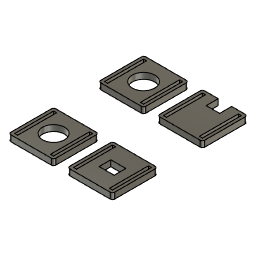
Bracelets v2 (Autodesk Fusion 360 design; units mm, degrees)
Autodesk Fusion 360 part; units mm, degrees
ref_plane "WorkPlane1" through (0, 0, 0) normal (0, 0, 1) x (1, 0, 0)
sketch "Sketch1" plane through (0, 0, 0) normal (0, 0, 1) x (1, 0, 0)
  line L0 (1.5, 0) -> (28.5, 0)
  line L1 (30, 1.5) -> (30, 28.5)
  line L2 (28.5, 30) -> (1.5, 30)
  line L3 (0, 28.5) -> (0, 1.5)
  arc A0 (30, 28.5) -> (28.5, 30) centre (28.5, 28.5) ccw
  arc A1 (1.5, 30) -> (0, 28.5) centre (1.5, 28.5) ccw
  arc A2 (0, 1.5) -> (1.5, 0) centre (1.5, 1.5) ccw
  arc A3 (28.5, 0) -> (30, 1.5) centre (28.5, 1.5) ccw
  line L4 (15, 0) -> (15, 30) construction
  line L5 (34.631, -0.4878) -> (34.631, 26.5001) construction
  line L6 (30, 15) -> (0, 15) construction
  arc A4 (40.762, 30) -> (39.262, 28.5) centre (40.762, 28.5) ccw
  line L7 (40.762, 30) -> (67.762, 30)
  arc A5 (69.262, 28.5) -> (67.762, 30) centre (67.762, 28.5) ccw
  line L8 (69.262, 28.5) -> (69.262, 1.5)
  arc A6 (67.762, 0) -> (69.262, 1.5) centre (67.762, 1.5) ccw
  line L9 (67.762, 0) -> (40.762, 0)
  arc A7 (39.262, 1.5) -> (40.762, 0) centre (40.762, 1.5) ccw
  line L10 (39.262, 1.5) -> (39.262, 28.5)
  line L11 (39.262, 15) -> (69.262, 15) construction
  line L12 (54.262, 0) -> (54.262, 30) construction
  line L13 (4, 2) -> (2, 2)
  line L14 (2, 2) -> (2, 28)
  line L15 (2, 28) -> (4, 28)
  line L16 (4, 28) -> (4, 2)
  line L17 (28, 28) -> (26, 28)
  line L18 (26, 28) -> (26, 2)
  line L19 (28, 2) -> (28, 28)
  line L20 (26, 2) -> (28, 2)
  line L21 (67.262, 28) -> (65.262, 28)
  line L22 (65.262, 28) -> (65.262, 2)
  line L23 (67.262, 2) -> (67.262, 28)
  line L24 (65.262, 2) -> (67.262, 2)
  line L25 (43.262, 28) -> (43.262, 2)
  line L26 (41.262, 2) -> (41.262, 28)
  line L27 (43.262, 2) -> (41.262, 2)
  line L28 (41.262, 28) -> (43.262, 28)
  line L29 (0, 45) -> (70, 45) construction
  line L30 (67.262, 62) -> (65.262, 62)
  line L31 (43.262, 62) -> (43.262, 88)
  line L32 (28, 88) -> (28, 62)
  arc A8 (28.5, 60) -> (30, 61.5) centre (28.5, 61.5) ccw
  line L33 (34.631, 90.4878) -> (34.631, 63.4999) construction
  line L34 (4, 88) -> (2, 88)
  line L35 (15, 90) -> (15, 60) construction
  line L36 (39.262, 75) -> (69.262, 75) construction
  arc A9 (40.762, 90) -> (39.262, 88.5) centre (40.762, 88.5) ccw
  arc A10 (30, 88.5) -> (28.5, 90) centre (28.5, 88.5) ccw
  arc A11 (67.762, 60) -> (69.262, 61.5) centre (67.762, 61.5) ccw
  line L37 (0, 61.5) -> (0, 88.5)
  line L38 (30, 88.5) -> (30, 61.5)
  line L39 (1.5, 90) -> (28.5, 90)
  arc A12 (1.5, 90) -> (0, 88.5) centre (1.5, 88.5) ccw
  line L40 (4, 62) -> (4, 88)
  line L41 (28, 62) -> (26, 62)
  arc A13 (39.262, 61.5) -> (40.762, 60) centre (40.762, 61.5) ccw
  line L42 (65.262, 88) -> (67.262, 88)
  line L43 (26, 88) -> (28, 88)
  line L44 (65.262, 62) -> (65.262, 88)
  line L45 (41.262, 62) -> (43.262, 62)
  line L46 (67.262, 88) -> (67.262, 62)
  line L47 (2, 88) -> (2, 62)
  line L48 (2, 62) -> (4, 62)
  line L49 (67.762, 90) -> (40.762, 90)
  line L50 (69.262, 61.5) -> (69.262, 88.5)
  arc A14 (0, 61.5) -> (1.5, 60) centre (1.5, 61.5) ccw
  line L51 (40.762, 60) -> (67.762, 60)
  line L52 (41.262, 88) -> (41.262, 62)
  line L53 (28.5, 60) -> (1.5, 60)
  line L54 (30, 75) -> (0, 75) construction
  line L55 (54.262, 90) -> (54.262, 60) construction
  line L56 (43.262, 88) -> (41.262, 88)
  arc A15 (69.262, 88.5) -> (67.762, 90) centre (67.762, 88.5) ccw
  line L57 (26, 62) -> (26, 88)
  line L58 (39.262, 88.5) -> (39.262, 61.5)
  circle A16 centre (15, 15) radius 7.3
  circle A17 centre (15, 75) radius 7.5
  line L59 (59.262, 18.9) -> (49.262, 18.9)
  line L60 (49.262, 18.9) -> (49.262, 11.1)
  line L61 (49.262, 11.1) -> (59.262, 11.1)
  line L62 (59.262, 11.1) -> (59.262, 18.9)
  line L63 (59.262, 18.9) -> (49.262, 11.1) construction
  line L64 (49.262, 18.9) -> (59.262, 11.1) construction
  line L65 (49.762, 82) -> (58.762, 82)
  line L66 (15, 82.5) -> (61.4441, 82.5) construction
  line L67 (49.762, 82) -> (49.762, 90)
  line L68 (58.762, 82) -> (58.762, 90)
  line L69 (58.762, 90) -> (49.762, 90)
  point P0 (30, 0)
  point P1 (0, 30)
  point P2 (0, 90)
  point P3 (0, 60)
  point P4 (30, 90)
  point P5 (0, 90)
  point P6 (54.262, 15)
  dimension "d9" = 30
  dimension "d10" = 30
  dimension "d18" = 1.5
  dimension "d19" = 1.5
  dimension "d20" = 1.5
  dimension "d21" = 1.5
  dimension "d41" = 2
  dimension "d42" = 2
  dimension "d43" = 2
  dimension "d44" = 2
  dimension "d45" = 14.6
  dimension "d46" = 15
  dimension "d54" = 10
  dimension "d55" = 7.8
  dimension "d57" = 9
  constraint horizontal L0
  constraint vertical L1
  constraint horizontal L2
  constraint vertical L3
  constraint tangent L1 A0
  constraint tangent L2 A0
  constraint coincident P1 L2
  constraint coincident P1 L3
  constraint tangent L2 A1
  constraint tangent L3 A1
  constraint coincident origin L0
  constraint coincident origin L3
  constraint tangent L0 A2
  constraint tangent L3 A2
  constraint coincident P0 L0
  constraint coincident P0 L1
  constraint tangent L0 A3
  constraint tangent L1 A3
  constraint midpoint L0 L4.start
  constraint midpoint L2 L4.end
  constraint midpoint L1 L6.start
  constraint midpoint L3 L6.end
  constraint symmetric L1.end L5 A4.end
  constraint symmetric L2.start L5 A4.start
  constraint symmetric A0 L5 A4
  constraint symmetric L2.end L5 L7.end
  constraint symmetric L3.start L5 A5.start
  constraint symmetric A1 L5 A5
  constraint symmetric L0.start L5 A6.start
  constraint symmetric L3.end L5 L8.end
  constraint symmetric A2 L5 A6
  constraint symmetric L0.end L5 L9.end
  constraint symmetric L1.start L5 A7.start
  constraint symmetric A3 L5 A7
  constraint symmetric L4.start L5 L12.start
  constraint symmetric L4.end L5 L12.end
  constraint symmetric L5 L6.start L11.start
  constraint symmetric L5 L6.end L11.end
  constraint parallel L4 L5
  constraint horizontal L13
  constraint vertical L14
  constraint horizontal L15
  constraint vertical L16
  constraint symmetric L4 L13.start L18.end
  constraint symmetric L4 L13.end L19.start
  constraint symmetric L4 L14.end L17.start
  constraint symmetric L4 L15.end L17.end
  constraint symmetric L5 L13.start L22.end
  constraint symmetric L5 L13.end L23.start
  constraint symmetric L5 L14.end L21.start
  constraint symmetric L5 L15.end L21.end
  constraint symmetric L5 L17.start L26.end
  constraint symmetric L5 L17.end L25.start
  constraint symmetric L5 L18.end L25.end
  constraint symmetric L5 L19.start L26.start
  constraint horizontal L29
  constraint symmetric origin L29 P5
  constraint symmetric P0 L29 P4
  constraint symmetric P1 L29 P3
  constraint symmetric L1.end L29 A8.end
  constraint symmetric L2.start L29 A8.start
  constraint symmetric A0 L29 A8
  constraint symmetric L2.end L29 A14.end
  constraint symmetric L3.start L29 L37.start
  constraint symmetric A1 L29 A14
  constraint symmetric L0.start L29 L39.start
  constraint symmetric L3.end L29 L37.end
  constraint symmetric A2 L29 A12
  constraint symmetric L0.end L29 A10.end
  constraint symmetric L1.start L29 A10.start
  constraint symmetric A3 L29 A10
  constraint symmetric L4.start L29 L35.start
  constraint symmetric L4.end L29 L35.end
  constraint symmetric L5.start L29 L33.start
  constraint symmetric L5.end L29 L33.end
  constraint symmetric L6.start L29 L54.start
  constraint symmetric L6.end L29 L54.end
  constraint symmetric A4.end L29 A13.start
  constraint symmetric A4.start L29 A13.end
  constraint symmetric A4 L29 A13
  constraint symmetric L7.end L29 A11.start
  constraint symmetric A5.start L29 A11.end
  constraint symmetric A5 L29 A11
  constraint symmetric L8.end L29 L50.end
  constraint symmetric A6.start L29 L49.start
  constraint symmetric A6 L29 A15
  constraint symmetric L9.end L29 A9.start
  constraint symmetric A7.start L29 A9.end
  constraint symmetric A7 L29 A9
  constraint symmetric L11.start L29 L36.start
  constraint symmetric L11.end L29 L36.end
  constraint symmetric L12.start L29 L55.start
  constraint symmetric L12.end L29 L55.end
  constraint symmetric L13.start L29 L34.start
  constraint symmetric L13.end L29 L34.end
  constraint symmetric L14.end L29 L47.end
  constraint symmetric L15.end L29 L40.start
  constraint symmetric L17.start L29 L32.end
  constraint symmetric L17.end L29 L41.end
  constraint symmetric L18.end L29 L43.start
  constraint symmetric L19.start L29 L32.start
  constraint symmetric L21.start L29 L30.start
  constraint symmetric L21.end L29 L30.end
  constraint symmetric L22.end L29 L42.start
  constraint symmetric L23.start L29 L42.end
  constraint symmetric L25.start L29 L31.start
  constraint symmetric L25.end L29 L31.end
  constraint symmetric L26.start L29 L52.start
  constraint symmetric L26.end L29 L45.start
  constraint midpoint L4 A16.centre
  constraint midpoint L54 A17.centre
  constraint horizontal L59
  constraint perpendicular L59 L60
  constraint parallel L59 L61
  constraint parallel L60 L62
  constraint coincident L63 P6
  constraint coincident L64 P6
  constraint midpoint L11 P6
  constraint perpendicular L55 L65
  constraint coincident A17 L66.start
  constraint coincident L35 L66.start
  constraint tangent A17 L66
  constraint coincident L49 L67.end
  constraint perpendicular L49 L67
  constraint coincident L49 L68.end
  constraint perpendicular L49 L68
  measures "d9" distance of origin P0
  measures "d10" distance of origin P1
  measures "d18" radius of A0
  measures "d19" radius of A1
  measures "d20" radius of A2
  measures "d21" radius of A3
  measures "d41" distance of L2 L15
  measures "d42" distance of L0 L13
  measures "d43" distance of L14.end L15.end
  measures "d44" distance of L3 L14
  measures "d45" diameter of A16
  measures "d46" diameter of A17
  measures "d54" distance of L60.end L61.end
  measures "d55" distance of L59.end L60.end
  measures "d57" distance of L65.start L65.end
extrude "Extrude4" add sketch "Sketch1" along normal blind 4 contours L0 L1 L2 L3 A0 A1 A2 A3 | A4 L7 A5 L8 A6 L9 A7 L10 | A8 A10 L37 L38 L39 A12 A14 L53 | A9 A11 A13 L49 L50 L51 A15 L58 L65 L67 L68 makes body 1 at (14.8182, 26.0932, 0) makes body 2 at (15.1868, 63.8403, 0) makes body 3 at (52.5953, 5.0333, 0) makes body 4 at (55.762, 68.6667, 0)
sketch "speaker_top" plane through (0, 0, 4) normal (0, 0, 1) x (-1, 0, 0)
  circle A0 centre (-15, -75) radius 7.5
  line L0 (-28, -62) -> (-26, -62)
  line L1 (-26, -62) -> (-26, -88)
  line L2 (-26, -88) -> (-28, -88)
  line L3 (-28, -88) -> (-28, -62)
  line L4 (-4, -62) -> (-2, -62)
  line L5 (-2, -62) -> (-2, -88)
  line L6 (-2, -88) -> (-4, -88)
  line L7 (-4, -88) -> (-4, -62)
  arc A1 (-30, -88.5) -> (-28.5, -90) centre (-28.5, -88.5) ccw
  line L8 (-28.5, -90) -> (-1.5, -90)
  arc A2 (-1.5, -90) -> (0, -88.5) centre (-1.5, -88.5) ccw
  line L9 (0, -88.5) -> (0, -61.5)
  arc A3 (0, -61.5) -> (-1.5, -60) centre (-1.5, -61.5) ccw
  line L10 (-1.5, -60) -> (-28.5, -60)
  arc A4 (-28.5, -60) -> (-30, -61.5) centre (-28.5, -61.5) ccw
  line L11 (-30, -61.5) -> (-30, -88.5)
sketch "speaker_bottom" plane through (0, 0, 4) normal (0, 0, 1) x (-1, 0, 0)
  line L0 (-41.262, -88) -> (-43.262, -88)
  line L1 (-43.262, -88) -> (-43.262, -62)
  line L2 (-43.262, -62) -> (-41.262, -62)
  line L3 (-41.262, -62) -> (-41.262, -88)
  line L4 (-65.262, -88) -> (-67.262, -88)
  line L5 (-67.262, -88) -> (-67.262, -62)
  line L6 (-67.262, -62) -> (-65.262, -62)
  line L7 (-65.262, -62) -> (-65.262, -88)
  line L8 (-49.762, -82) -> (-49.762, -90)
  line L9 (-49.762, -90) -> (-40.762, -90)
  arc A0 (-40.762, -90) -> (-39.262, -88.5) centre (-40.762, -88.5) ccw
  line L10 (-39.262, -88.5) -> (-39.262, -61.5)
  arc A1 (-39.262, -61.5) -> (-40.762, -60) centre (-40.762, -61.5) ccw
  line L11 (-40.762, -60) -> (-67.762, -60)
  arc A2 (-67.762, -60) -> (-69.262, -61.5) centre (-67.762, -61.5) ccw
  line L12 (-69.262, -61.5) -> (-69.262, -88.5)
  arc A3 (-69.262, -88.5) -> (-67.762, -90) centre (-67.762, -88.5) ccw
  line L13 (-67.762, -90) -> (-58.762, -90)
  line L14 (-58.762, -90) -> (-58.762, -82)
  line L15 (-58.762, -82) -> (-49.762, -82)
sketch "mic_top" plane through (0, 0, 4) normal (0, 0, 1) x (-1, 0, 0)
  circle A0 centre (-15, -15) radius 7.3
  line L0 (-28, -2) -> (-26, -2)
  line L1 (-26, -2) -> (-26, -28)
  line L2 (-26, -28) -> (-28, -28)
  line L3 (-28, -28) -> (-28, -2)
  line L4 (-2, -28) -> (-4, -28)
  line L5 (-4, -28) -> (-4, -2)
  line L6 (-4, -2) -> (-2, -2)
  line L7 (-2, -2) -> (-2, -28)
  arc A1 (-28.5, 0) -> (-30, -1.5) centre (-28.5, -1.5) ccw
  line L8 (-30, -1.5) -> (-30, -28.5)
  arc A2 (-30, -28.5) -> (-28.5, -30) centre (-28.5, -28.5) ccw
  line L9 (-28.5, -30) -> (-1.5, -30)
  arc A3 (-1.5, -30) -> (0, -28.5) centre (-1.5, -28.5) ccw
  line L10 (0, -28.5) -> (0, -1.5)
  arc A4 (0, -1.5) -> (-1.5, 0) centre (-1.5, -1.5) ccw
  line L11 (-1.5, 0) -> (-28.5, 0)
sketch "mic_bottom" plane through (0, 0, 4) normal (0, 0, 1) x (-1, 0, 0)
  line L0 (-67.262, -2) -> (-65.262, -2)
  line L1 (-65.262, -2) -> (-65.262, -28)
  line L2 (-65.262, -28) -> (-67.262, -28)
  line L3 (-67.262, -28) -> (-67.262, -2)
  line L4 (-41.262, -2) -> (-41.262, -28)
  line L5 (-41.262, -28) -> (-43.262, -28)
  line L6 (-43.262, -28) -> (-43.262, -2)
  line L7 (-43.262, -2) -> (-41.262, -2)
  line L8 (-59.262, -18.9) -> (-59.262, -11.1)
  line L9 (-59.262, -11.1) -> (-49.262, -11.1)
  line L10 (-49.262, -11.1) -> (-49.262, -18.9)
  line L11 (-49.262, -18.9) -> (-59.262, -18.9)
  arc A0 (-67.762, 0) -> (-69.262, -1.5) centre (-67.762, -1.5) ccw
  line L12 (-69.262, -1.5) -> (-69.262, -28.5)
  arc A1 (-69.262, -28.5) -> (-67.762, -30) centre (-67.762, -28.5) ccw
  line L13 (-67.762, -30) -> (-40.762, -30)
  arc A2 (-40.762, -30) -> (-39.262, -28.5) centre (-40.762, -28.5) ccw
  line L14 (-39.262, -28.5) -> (-39.262, -1.5)
  arc A3 (-39.262, -1.5) -> (-40.762, 0) centre (-40.762, -1.5) ccw
  line L15 (-40.762, 0) -> (-67.762, 0)
equation "microphone_diameter = 14.6 mm"
equation "speaker_diameter = 15 mm"
equation "object_length = 30 mm"
equation "object_height = 4 mm"
equation "tolerance_to_object = 2 mm"
equation "strap_height = 25 mm"
equation "strap_width = 2 mm"
equation "d9 = object_length"
equation "d10 = object_length"
equation "d41 = tolerance_to_object"
equation "d42 = tolerance_to_object"
equation "d43 = strap_width"
equation "d44 = tolerance_to_object"
equation "d45 = microphone_diameter"
equation "d46 = speaker_diameter"
equation "speaker_connector_distance = 9 mm"
equation "mic_connector_distance = 10 mm"
equation "d54 = mic_connector_distance"
equation "d55 = mic_pin_length"
equation "mic_pin_length = 7.8 mm"
equation "d57 = speaker_connector_distance"
equation "d60 = object_height"
